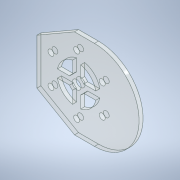
# Autodesk Inventor part: Standalone_Valve_Base_Plate
Saved by Autodesk Inventor 2020 (Build 240168000, 168)
## iProperties
Created: 2021-07-01
Part Number: Standalone_Valve_Base_Plate
Material: Glass
Document SubType Name: Modeling
Designer: Workshop
Density: 2.18 g/cm^3
Appearance: Clear
Author: Workshop
Autodesk Inventor part; units mm, degrees
ref_plane "YZ Plane" through (0, 0, 0) normal (1, 0, 0) x (0, 1, 0)
ref_plane "XZ Plane" through (0, 0, 0) normal (0, 1, 0) x (-1, 0, 0)
ref_plane "XY Plane" through (0, 0, 0) normal (0, 0, 1) x (1, 0, 0)
sketch "Sketch1" plane through (0, 0, 0) normal (0, 0, 1) x (1, 0, 0)
  arc A0 (9, -22.4752) -> (8.9991, 22.4772) centre (8.9998, 0.001) ccw projected
  line L0 (8.9991, 22.4772) -> (-1.0724, 22.4739) projected
  line L1 (-1.0724, 22.4739) -> (-20, 11.546) projected
  line L2 (-20, 11.546) -> (-20, -11.548) projected
  line L3 (-20, -11.548) -> (-1.0716, -22.4763) projected
  line L4 (-1.0716, -22.4763) -> (9, -22.4752) projected
  line L5 (2.052, 3.5186) -> (2.052, 9.6538) projected
  arc A1 (9.6607, 2.019) -> (2.052, 9.6538) centre (0, 0) ccw projected
  line L6 (9.6607, 2.019) -> (3.5411, 2.0129) projected
  arc A2 (3.5411, 2.0129) -> (2.052, 3.5186) centre (0, 0) ccw projected
  line L7 (2.052, -3.5186) -> (2.052, -9.6538) projected
  arc A3 (2.052, -9.6538) -> (9.6607, -2.019) centre (0, 0) ccw projected
  line L8 (9.6607, -2.019) -> (3.5411, -2.0129) projected
  arc A4 (2.052, -3.5186) -> (3.5411, -2.0129) centre (0, 0) ccw projected
  circle A5 centre (12.9254, 7.4625) radius 1.5 projected
  circle A6 centre (12.9254, 7.4625) radius 1.5 projected
  circle A7 centre (12.9254, -7.4625) radius 1.5 projected
  circle A8 centre (12.9254, -7.4625) radius 1.5 projected
  circle A9 centre (0, -14.925) radius 1.5 projected
  circle A10 centre (0, -14.925) radius 1.5 projected
  circle A11 centre (0, 14.925) radius 1.5 projected
  circle A12 centre (0, 0) radius 2.25 projected
  line L9 (-2.052, -3.5186) -> (-2.052, -9.6538) projected
  arc A13 (-9.6607, -2.019) -> (-2.052, -9.6538) centre (0, 0) ccw projected
  line L10 (-9.6607, -2.019) -> (-3.5411, -2.0129) projected
  arc A14 (-3.5411, -2.0129) -> (-2.052, -3.5186) centre (0, 0) ccw projected
  line L11 (-2.052, 3.5186) -> (-2.052, 9.6538) projected
  arc A15 (-2.052, 9.6538) -> (-9.6607, 2.019) centre (0, 0) ccw projected
  line L12 (-9.6607, 2.019) -> (-3.5411, 2.0129) projected
  arc A16 (-2.052, 3.5186) -> (-3.5411, 2.0129) centre (0, 0) ccw projected
  circle A17 centre (-12.9254, -7.4625) radius 1.5 projected
  circle A18 centre (-12.9254, -7.4625) radius 1.5 projected
  circle A19 centre (-12.9254, 7.4625) radius 1.5 projected
  circle A20 centre (-12.9254, 7.4625) radius 1.5 projected
  circle A21 centre (0, 14.925) radius 1.5 projected
  point P0 (0, 0)
extrude "Extrusion1" add sketch "Sketch1" along normal mid plane 2
body "Solid1"
